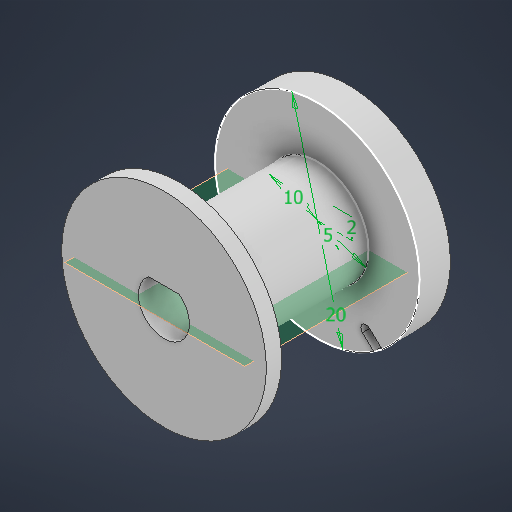
# Autodesk Inventor part: D_coupler
Saved by Autodesk Inventor 2027 (Build 310192000, 192)
## iProperties
Created: 2026-05-09
Part Number: D_coupler
Material: Generic
Document SubType Name: Modeling
Designer: alexy
Density: 1 g/cm^3
Appearance: Default
Author: alexy
Autodesk Inventor part; units mm, degrees
ref_plane "YZ Plane" through (0, 0, 0) normal (1, 0, 0) x (0, 1, 0)
ref_plane "XZ Plane" through (0, 0, 0) normal (0, 1, 0) x (-1, 0, 0)
ref_plane "XY Plane" through (0, 0, 0) normal (0, 0, 1) x (1, 0, 0)
sketch "Sketch1" plane through (0, 0, 0) normal (0, 0, 1) x (1, 0, 0)
  circle A0 centre (0, 0) radius 2.5
  line L0 (-1.5, 2) -> (1.5, 2)
  circle A1 centre (0, 0) radius 5
  circle A2 centre (0, 0) radius 10
  dimension "d0" = 5
  dimension "d1" = 2
  dimension "d2" = 10
  dimension "d16" = 20
  constraints: 3 centre point, 3 coincident, 2 end point, 2 point on circle, 1 horizontal
  measures "d0" diameter of A0
  measures "d1" distance from line of point (0, 0) L0
  measures "d2" diameter of A1
  measures "d16" diameter of A2
extrude "Extrusion1" add sketch "Sketch1" along normal blind 15 contours L0 A0 | A1 picked at (-0.3466, 2.0912)
extrude "Extrusion2" add sketch "Sketch1" against normal blind 3 contours L0 A0 | A1 | A2 picked at (-0.3466, 2.0912)
ref_plane "Work Plane2" through (0, 0, 0) normal (0, -1, 0) x (1, 0, 0)
ref_plane "Work Plane1" through (0, 5, 0) normal (0, -1, 0) x (1, 0, 0)
sketch "Sketch4" plane through (0, 0, 0) normal (0, -1, 0) x (1, 0, 0)
  line L0 (5, 15) -> (-5, 15) projected
  line L1 (-5, 15) -> (-10, 15)
  line L2 (-10, 15) -> (-10, 13.5)
  line L3 (-5, 0) -> (-5, 15) projected
  line L4 (-10, 13.5) -> (-5, 10.1834)
  line L5 (0, -6.6) -> (0, 18.6) projected
  point P0 (0, 0)
  dimension "d10" = 5
  dimension "d11" = 1.5
  dimension "d14" = 6
  constraints: 6 end point, 1 horizontal, 1 point on line, 1 vertical
  measures "d10" distance of L0.end L1.end
  measures "d11" distance of L1.end L2.end
  measures "d14" distance of L2.end L4.end
revolve "Revolution1" add sketch "Sketch4" angle 360 about axis through (0, 0, -10) along (0, 0, 1)
sketch "Sketch6" plane through (0, 0, -3) normal (0, 0, -1) x (-1, 0, 0)
  circle A0 centre (0, 0) radius 10 projected
  circle A1 centre (-4.7517, -6.9277) radius 0.5
  line L0 (-5.0949, -6.5641) -> (-6.3365, -7.7362)
  line L1 (-4.4085, -7.2913) -> (-5.5187, -8.3393)
  dimension "d19" = 1
  constraints: 4 end point, 4 point on circle, 2 tangent, 1 centre point, 1 parallel
  measures "d19" diameter of A1
extrude "Extrusion3" cut sketch "Sketch6" against normal blind 3 contours L0 A1 L1 A0 | A1 picked at (-5.8735, -7.6008)
body "Solid1"
